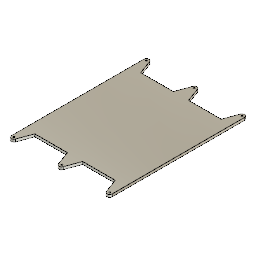
1-Cold Build Plate v1 (Autodesk Fusion 360 design; units mm, degrees)
Autodesk Fusion 360 part; units mm, degrees
mesh "Mesh1" [no effect]
sketch "Mesh Selection Sketch XY" plane through (0, 0, 5) normal (0, 0, 1) x (1, 0, 0)
sketch "Sketch2" plane through (0, 0, 0) normal (0, 0, 1) x (1, 0, 0)
  line L0 (190.5, -260) -> (-190.5, -260)
  line L1 (-190.5, -260) -> (-190.5, 260)
  line L2 (-190.5, 260) -> (190.5, 260)
  line L3 (190.5, 260) -> (190.5, -260)
  line L4 (190.5, -260) -> (-190.5, 260) construction
  line L5 (-190.5, -260) -> (190.5, 260) construction
  line L6 (-151.5, 200) -> (151.5, 200)
  line L7 (151.5, 200) -> (151.5, -200)
  line L8 (151.5, -200) -> (-151.5, -200)
  line L9 (-151.5, -200) -> (-151.5, 200)
  line L10 (-151.5, 200) -> (151.5, -200) construction
  line L11 (151.5, 200) -> (-151.5, -200) construction
  circle A0 centre (-180.5, 250) radius 2.75
  line L12 (-171.1184, 253.462) -> (-151.5, 200)
  circle A1 centre (0, 250) radius 2.75
  circle A2 centre (180.5, 250) radius 2.75
  circle A3 centre (-180.5, -250) radius 2.75
  circle A4 centre (0, -250) radius 2.75
  circle A5 centre (180.5, -250) radius 2.75
  arc A6 (-170.5, 250) -> (-190.5, 250) centre (-180.5, 250) ccw
  line L13 (-180.5, 250) -> (-170.5, 250) construction
  line L14 (-180.5, 250) -> (-190.5, 250) construction
  arc A7 (10, 250) -> (-10, 250) centre (0, 250) ccw
  arc A8 (190.5, 250) -> (170.5, 250) centre (180.5, 250) ccw
  line L15 (-29, 200) -> (-9.3879, 253.445)
  line L16 (9.3879, 253.445) -> (29, 200)
  line L17 (20, 0) -> (2.5, 0)
  line L18 (151.5, 200) -> (171.1121, 253.445)
  line L19 (-171.1184, -253.462) -> (-151.5, -200)
  arc A9 (-190.5, -250) -> (-170.5, -250) centre (-180.5, -250) ccw
  line L20 (-29, -200) -> (-9.3879, -253.445)
  line L21 (9.3879, -253.445) -> (29, -200)
  arc A10 (-10, -250) -> (10, -250) centre (0, -250) ccw
  line L22 (151.5, -200) -> (171.1121, -253.445)
  arc A11 (170.5, -250) -> (190.5, -250) centre (180.5, -250) ccw
  dimension "d1" = 381
  dimension "d2" = 520
  dimension "d3" = 400
  dimension "d4" = 303
  dimension "d5" = 5.5
  dimension "d6" = 10
  dimension "d7" = 10
  dimension "d10" = 361
  dimension "d11" = -500
  dimension "d12" = 180
  dimension "d13" = 110.151
  dimension "d14" = 110.151
  constraint perpendicular L0 L1
  constraint parallel L0 L2
  constraint parallel L1 L3
  constraint horizontal L0
  constraint coincident L4 origin
  constraint coincident L5 origin
  constraint perpendicular L6 L7
  constraint parallel L6 L8
  constraint parallel L7 L9
  constraint horizontal L6
  constraint coincident L10 origin
  constraint coincident L11 origin
  constraint coincident L1 A6.end
  constraint coincident A0.centre A6.centre
  constraint tangent L12 A6
  constraint coincident L6 L15.start
  constraint coincident A7 L15.end
  constraint coincident A7 L16.start
  constraint coincident L6 L16.end
  constraint tangent A7 L16
  constraint tangent A7 L15
  constraint equal L15 L16
  constraint coincident A8 L18.end
  constraint tangent A8 L18
  constraint horizontal L13
  constraint symmetric L6.start L17 L8.end
  constraint symmetric L6.end L17 L7.end
  constraint symmetric L12.start L17 L19.start
  constraint symmetric A6.start L17 A9.end
  constraint symmetric A6.end L17 A9.start
  constraint symmetric A6 L17 A9
  constraint symmetric A7.start L17 A10.end
  constraint symmetric A7.end L17 A10.start
  constraint symmetric A7 L17 A10
  constraint symmetric A8.start L17 A11.end
  constraint symmetric A8.end L17 A11.start
  constraint symmetric A8 L17 A11
  constraint symmetric L15.start L17 L20.start
  constraint symmetric L15.end L17 L20.end
  constraint symmetric L16.start L17 L21.start
  constraint symmetric L16.end L17 L21.end
  constraint symmetric L17 L18.end L22.end
  measures "d1" distance of L0.start L0.end
  measures "d2" distance of L0.end L1.end
  measures "d3" distance of L6.start L8.end
  measures "d4" distance of L7.end L8.end
  measures "d5" diameter of A0
  measures "d6" distance of L1 A0.centre A1.centre
  measures "d7" distance of L2 A0.centre A1.centre
  measures "d12" angle of L13 L14
  measures "d13" angle of L6 L12
  measures "d14" angle of L6 L15
extrude "Extrude1" add sketch "Sketch2" along normal blind 10 contours L3 L7 A8 L18 L22 A11 | L8 L20 L21 A10 | L1 L9 L12 A6 L19 A9 | L6 L7 L8 L9 | L6 A7 L15 L16
